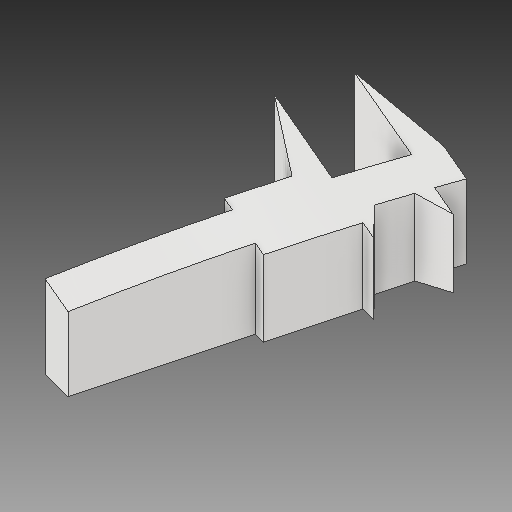
# Autodesk Inventor part: Team Pin Cad-Caliper
Saved by Autodesk Inventor 2017 (Build 210142000, 142)
## iProperties
Created: 2016-02-20
Part Number: Team Pin Cad-Caliper
Material: Generic
Document SubType Name: Modeling
Designer: RoksBot
Density: 1 g/cm^3
Appearance: White
Author: RoksBot
Autodesk Inventor part; units mm, degrees
ref_plane "YZ Plane" through (0, 0, 0) normal (1, 0, 0) x (0, 1, 0)
ref_plane "XZ Plane" through (0, 0, 0) normal (0, 1, 0) x (-1, 0, 0)
ref_plane "XY Plane" through (0, 0, 0) normal (0, 0, 1) x (1, 0, 0)
sketch "Sketch1" plane through (0, 0, 0) normal (0, 0, 1) x (1, 0, 0)
  line L0 (0, 0) -> (0, 8.6646) construction
  line L1 (20.9931, 1.27) -> (20.9931, 5.715)
  line L2 (20.9931, 5.715) -> (27.9781, 3.81)
  line L3 (27.9781, 3.81) -> (27.9781, 0)
  line L4 (27.9781, 0) -> (20.9931, 0)
  line L5 (20.9931, 1.27) -> (18.4531, 1.27)
  line L6 (18.4531, 1.27) -> (18.4531, 0)
  line L7 (18.4531, 0) -> (20.9931, 0)
  dimension "d0" = 20.9931
  dimension "d1" = 4.445
  dimension "d2" = 1.27
  dimension "d3" = 2.54
  dimension "d4" = 3.81
  dimension "d5" = 6.985
  constraints: 16 end point, 2 parallel, 2 perpendicular, 2 vertical, 1 horizontal, 1 horizontal alignment
  measures "d0" distance between parallel lines of L0 L1
  measures "d1" distance from line of L5 L1.end
  measures "d2" distance of L5.end L6.end
  measures "d3" distance between parallel lines of L1 L6
  measures "d4" distance of L2.end L3.end
  measures "d5" distance between parallel lines of L1 L3
revolve "Revolution1" add sketch "Sketch1" angle 360 about axis through (0, 0, 0) along (0, 1, 0)
sketch "Sketch2" plane through (0, 1.27, 0) normal (0, 1, 0) x (1, 0, 0)
  circle A0 centre (0, 0) radius 20.9931 projected
  circle A1 centre (0, 0) radius 27.9781 projected
  circle A2 centre (0, 0) radius 18.4531 projected
  line L0 (-4.2505, -7.1349) -> (4.1315, -7.1349) projected
  circle A3 centre (0, 0) radius 19.685 projected
  line L1 (-12.7595, -2.2222) -> (-12.7595, -29.7716) construction
  line L2 (12.6405, -2.2222) -> (12.6405, -30.8961) construction
  line L3 (-12.7549, -7.1349) -> (-31.6502, -7.1349) construction
  line L4 (0, 0) -> (17.3317, 30.0193) construction
  line L5 (-18.5741, 9.7833) -> (-25.4, 9.7833)
  line L6 (-18.8949, 9.1483) -> (-25.4, 9.1483)
  line L7 (-25.4, 9.1483) -> (-25.4, 9.7833)
  line L8 (-19.8553, -6.8174) -> (-25.4, -6.8174)
  line L9 (-25.4, -6.8174) -> (-25.4, -7.4524)
  line L10 (-25.4, -7.4524) -> (-19.6258, -7.4524)
  line L11 (0.1351, 9.4658) -> (-31.517, 9.4658) construction
  line L12 (-24.13, 9.1483) -> (-22.86, 6.9486)
  line L13 (-22.86, 6.9486) -> (-25.4, 6.9486)
  line L14 (-25.4, 6.9486) -> (-24.13, 9.1483)
  line L15 (-24.13, -6.8174) -> (-25.4, -4.6177)
  line L16 (-25.4, -4.6177) -> (-22.86, -4.6177)
  line L17 (-22.86, -4.6177) -> (-24.13, -6.8174)
  line L18 (-29.0818, 1.1654) -> (-16.5563, 1.1654) construction
  line L19 (-24.13, 7.6818) -> (-24.13, -5.3509) construction
  line L20 (-23.8125, 2.4354) -> (-24.4475, 2.4354)
  line L21 (-24.4475, 2.4354) -> (-24.4475, 6.9486)
  line L22 (-24.4475, 6.9486) -> (-23.8125, 6.9486)
  line L23 (-23.8125, 6.9486) -> (-23.8125, 2.4354)
  line L24 (-23.8125, 2.4354) -> (-24.4475, 6.9486) construction
  line L25 (-24.4475, 2.4354) -> (-23.8125, 6.9486) construction
  line L26 (-23.8125, -0.1046) -> (-24.4475, -0.1046)
  line L27 (-24.4475, -0.1046) -> (-24.4475, -4.6177)
  line L28 (-24.4475, -4.6177) -> (-23.8125, -4.6177)
  line L29 (-23.8125, -4.6177) -> (-23.8125, -0.1046)
  line L30 (-23.8125, -0.1046) -> (-24.4475, -4.6177) construction
  line L31 (-24.4475, -0.1046) -> (-23.8125, -4.6177) construction
  line L32 (-13.077, -16.4226) -> (-13.077, -23.7886)
  line L33 (-13.077, -23.7886) -> (-12.442, -23.7886)
  line L34 (-12.442, -23.7886) -> (-12.442, -16.9088)
  line L35 (12.323, -16.9957) -> (12.323, -23.7886)
  line L36 (12.323, -23.7886) -> (12.958, -23.7886)
  line L37 (12.958, -23.7886) -> (12.958, -16.5167)
  line L38 (-12.442, -22.5186) -> (-10.2423, -21.2486)
  line L39 (-10.2423, -21.2486) -> (-10.2423, -23.7886)
  line L40 (-10.2423, -23.7886) -> (-12.442, -22.5186)
  line L41 (12.323, -22.5186) -> (10.1233, -23.7886)
  line L42 (10.1233, -23.7886) -> (10.1233, -21.2486)
  line L43 (10.1233, -21.2486) -> (12.323, -22.5186)
  line L44 (-3.8695, -21.2486) -> (3.7505, -21.2486) construction
  line L45 (3.7505, -21.2486) -> (3.7505, -23.7886) construction
  line L46 (3.7505, -23.7886) -> (-3.8695, -23.7886) construction
  line L47 (-3.8695, -23.7886) -> (-3.8695, -21.2486) construction
  line L48 (-0.0595, -13.6296) -> (-0.0595, -32.797) construction
  line L49 (-10.2423, -22.5186) -> (10.1233, -22.5186) construction
  line L50 (-4.2505, -22.8361) -> (-10.2423, -22.8361)
  line L51 (-10.2423, -22.8361) -> (-10.2423, -22.2011)
  line L52 (-10.2423, -22.2011) -> (-4.2505, -22.2011)
  line L53 (-4.2505, -22.2011) -> (-4.2505, -22.8361)
  line L54 (-4.2505, -22.8361) -> (-10.2423, -22.2011) construction
  line L55 (-10.2423, -22.8361) -> (-4.2505, -22.2011) construction
  line L56 (4.1315, -22.2011) -> (10.1233, -22.2011)
  line L57 (10.1233, -22.2011) -> (10.1233, -22.8361)
  line L58 (10.1233, -22.8361) -> (4.1315, -22.8361)
  line L59 (4.1315, -22.8361) -> (4.1315, -22.2011)
  line L60 (4.1315, -22.2011) -> (10.1233, -22.8361) construction
  line L61 (10.1233, -22.2011) -> (4.1315, -22.8361) construction
  line L62 (10.2204, 18.3372) -> (11.1133, 19.8839)
  line L63 (11.1133, 19.8839) -> (11.6633, 19.5664)
  line L64 (11.6633, 19.5664) -> (10.7703, 18.0197)
  line L65 (12.8992, 20.8364) -> (18.6142, 20.8364) construction
  line L66 (18.6142, 20.8364) -> (18.6142, 18.2964) construction
  line L67 (18.6142, 18.2964) -> (12.8992, 18.2964) construction
  line L68 (12.8992, 18.2964) -> (12.8992, 20.8364) construction
  line L69 (11.1133, 19.8839) -> (12.8992, 19.8839)
  line L70 (12.8992, 19.8839) -> (12.8992, 19.2489)
  line L71 (12.8992, 19.2489) -> (11.1133, 19.2489)
  line L72 (11.1133, 19.2489) -> (11.1133, 19.8839)
  line L73 (11.1133, 19.8839) -> (12.8992, 19.2489) construction
  line L74 (12.8992, 19.8839) -> (11.1133, 19.2489) construction
  circle A4 centre (0, 0) radius 22.8981 construction
  line L75 (11.4654, -8.564) -> (6.3194, -8.564) projected
  spline S0 degree 2 poles (-4.3048, 23.0885) (-4.5009, 22.6771) (-4.9694, 22.2828) (-5.345, 22.1916) knots 0 0 0 1 2 2 2
  spline S1 degree 2 poles (-5.345, 22.1916) (-5.9856, 22.0361) (-6.5218, 22.4794) knots 0 0 0 1 1 1
  spline S2 degree 2 poles (-6.5218, 22.4794) (-7.071, 22.9258) (-7.2859, 23.8109) knots 0 0 0 1 1 1
  spline S3 degree 2 poles (-7.2859, 23.8109) (-7.5233, 24.7892) (-7.1789, 25.4155) knots 0 0 0 1 1 1
  spline S4 degree 2 poles (-7.1789, 25.4155) (-6.903, 25.9172) (-6.3614, 26.0486) knots 0 0 0 1 1 1
  spline S5 degree 2 poles (-6.3614, 26.0486) (-5.9392, 26.1511) (-5.6643, 26.0853) knots 0 0 0 1 1 1
  spline S6 degree 2 poles (-5.6643, 26.0853) (-5.3596, 26.0112) (-5.0862, 25.7107) knots 0 0 0 1 1 1
  spline S7 degree 2 poles (-5.0862, 25.7107) (-5.0278, 25.6478) (-5.0115, 25.5808) knots 0 0 0 1 1 1
  spline S8 degree 2 poles (-5.0115, 25.5808) (-4.9832, 25.4644) (-5.1191, 25.2618) (-5.2268, 25.2357) knots 0 0 0 1 2 2 2
  spline S9 degree 2 poles (-5.2268, 25.2357) (-5.3782, 25.1989) (-5.5051, 25.3408) knots 0 0 0 1 1 1
  spline S10 degree 2 poles (-5.5051, 25.3408) (-5.6451, 25.4856) (-5.8317, 25.5174) knots 0 0 0 1 1 1
  spline S11 degree 2 poles (-5.8317, 25.5174) (-5.9746, 25.5475) (-6.2279, 25.486) knots 0 0 0 1 1 1
  spline S12 degree 2 poles (-6.2279, 25.486) (-6.5569, 25.4061) (-6.7127, 25.0569) knots 0 0 0 1 1 1
  spline S13 degree 2 poles (-6.7127, 25.0569) (-6.906, 24.6338) (-6.7385, 23.9438) knots 0 0 0 1 1 1
  spline S14 degree 2 poles (-6.7385, 23.9438) (-6.5844, 23.309) (-5.8687, 22.6596) (-5.4727, 22.7557) knots 0 0 0 1 2 2 2
  spline S15 degree 2 poles (-5.4727, 22.7557) (-5.0447, 22.8596) (-4.8204, 23.3456) knots 0 0 0 1 1 1
  spline S16 degree 2 poles (-4.8204, 23.3456) (-4.7629, 23.4644) (-4.6377, 23.4948) knots 0 0 0 1 1 1
  spline S17 degree 2 poles (-4.6377, 23.4948) (-4.53, 23.521) (-4.3078, 23.393) (-4.2802, 23.2794) knots 0 0 0 1 2 2 2
  spline S18 degree 2 poles (-4.2802, 23.2794) (-4.2576, 23.1863) (-4.3048, 23.0885) knots 0 0 0 1 1 1
  spline S19 degree 2 poles (-2.5624, 23.1168) (-2.545, 22.971) (-2.7214, 22.7539) (-2.8582, 22.7376) knots 0 0 0 1 2 2 2
  spline S20 degree 2 poles (-2.8582, 22.7376) (-3.007, 22.7199) (-3.2201, 22.8877) (-3.2378, 23.0364) knots 0 0 0 1 2 2 2
  spline S21 degree 2 poles (-3.2378, 23.0364) (-3.254, 23.1733) (-3.087, 23.3923) (-2.9382, 23.41) knots 0 0 0 1 2 2 2
  spline S22 degree 2 poles (-2.9382, 23.41) (-2.8014, 23.4263) (-2.5783, 23.2507) (-2.5624, 23.1168) knots 0 0 0 1 2 2 2
  spline S23 degree 2 poles (1.6575, 23.2292) (1.6783, 23.1693) (1.6781, 23.1183) knots 0 0 0 1 1 1
  spline S24 degree 2 poles (1.6781, 23.1183) (1.6778, 22.9955) (1.4946, 22.8432) (1.3837, 22.8435) knots 0 0 0 1 2 2 2
  spline S25 degree 2 poles (1.3837, 22.8435) (1.189, 22.844) (1.1206, 23.024) knots 0 0 0 1 1 1
  line L76 (1.1206, 23.024) -> (0.9153, 23.5578)
  line L77 (0.9153, 23.5578) -> (-0.8255, 23.5626)
  line L78 (-0.8255, 23.5626) -> (-1.0307, 23.0328)
  spline S26 degree 2 poles (-1.0307, 23.0328) (-1.1001, 22.8503) (-1.2888, 22.8508) knots 0 0 0 1 1 1
  spline S27 degree 2 poles (-1.2888, 22.8508) (-1.4087, 22.8511) (-1.585, 23.0074) (-1.5847, 23.1272) knots 0 0 0 1 2 2 2
  spline S28 degree 2 poles (-1.5847, 23.1272) (-1.5846, 23.1812) (-1.5665, 23.2291) knots 0 0 0 1 1 1
  line L79 (-1.5665, 23.2291) -> (-0.2988, 26.5993)
  spline S29 degree 2 poles (-0.2988, 26.5993) (-0.2174, 26.8148) (0.0283, 26.8141) knots 0 0 0 1 1 1
  spline S30 degree 2 poles (0.0283, 26.8141) (0.28, 26.8135) (0.3484, 26.6245) knots 0 0 0 1 1 1
  line L80 (0.3484, 26.6245) -> (1.6575, 23.2292)
  line L81 (0.7221, 24.1366) -> (0.026, 25.9722)
  line L82 (0.026, 25.9722) -> (-0.6322, 24.1403)
  line L83 (-0.6322, 24.1403) -> (0.7221, 24.1366)
  spline S31 degree 2 poles (3.0603, 23.0562) (3.0422, 22.9105) (2.8189, 22.742) (2.6821, 22.7591) knots 0 0 0 1 2 2 2
  spline S32 degree 2 poles (2.6821, 22.7591) (2.5335, 22.7776) (2.3669, 22.9916) (2.3854, 23.1402) knots 0 0 0 1 2 2 2
  spline S33 degree 2 poles (2.3854, 23.1402) (2.4024, 23.277) (2.6172, 23.4495) (2.7658, 23.431) knots 0 0 0 1 2 2 2
  spline S34 degree 2 poles (2.7658, 23.431) (2.9026, 23.414) (3.077, 23.19) (3.0603, 23.0562) knots 0 0 0 1 2 2 2
  spline S35 degree 2 poles (7.2494, 23.9177) (6.9985, 22.8964) (6.3258, 22.4939) knots 0 0 0 1 1 1
  spline S36 degree 2 poles (6.3258, 22.4939) (5.7821, 22.1647) (5.1478, 22.3205) knots 0 0 0 1 1 1
  line L84 (5.1478, 22.3205) -> (4.1323, 22.5699)
  line L85 (4.1323, 22.5699) -> (5.0564, 26.3321)
  line L86 (5.0564, 26.3321) -> (6.069, 26.0834)
  spline S37 degree 2 poles (6.069, 26.0834) (6.6946, 25.9298) (7.047, 25.4051) knots 0 0 0 1 1 1
  spline S38 degree 2 poles (7.047, 25.4051) (7.4616, 24.7818) (7.2494, 23.9177) knots 0 0 0 1 1 1
  spline S39 degree 2 poles (6.7023, 24.052) (6.8474, 24.6427) (6.5732, 25.0587) knots 0 0 0 1 1 1
  spline S40 degree 2 poles (6.5732, 25.0587) (6.337, 25.416) (5.9267, 25.5167) knots 0 0 0 1 1 1
  line L87 (5.9267, 25.5167) -> (5.4641, 25.6304)
  line L88 (5.4641, 25.6304) -> (4.8173, 22.9971)
  line L89 (4.8173, 22.9971) -> (5.2857, 22.882)
  spline S41 degree 2 poles (5.2857, 22.882) (5.7047, 22.7791) (6.047, 22.9666) knots 0 0 0 1 1 1
  spline S42 degree 2 poles (6.047, 22.9666) (6.5215, 23.3159) (6.7023, 24.052) knots 0 0 0 1 1 1
  line L90 (-26.9128, 0.2129) -> (-27.3651, 0.2129)
  line L91 (-27.3651, 0.2129) -> (-27.3651, 0.7162)
  line L92 (-27.3651, 0.7162) -> (-26.9128, 0.7162)
  line L93 (-26.9128, 0.7162) -> (-26.9128, 0.2129)
  spline S43 degree 2 poles (-25.1468, 0.8613) (-25.1468, 0.5603) (-25.5281, 0.1728) (-25.8615, 0.1728) knots 0 0 0 1 2 2 2
  spline S44 degree 2 poles (-25.8615, 0.1728) (-26.0282, 0.1728) (-26.2891, 0.2685) (-26.3802, 0.3627) knots 0 0 0 1 2 2 2
  spline S45 degree 2 poles (-26.3802, 0.3627) (-26.4883, 0.4723) (-26.6041, 0.8196) (-26.6041, 1.062) knots 0 0 0 1 2 2 2
  spline S46 degree 2 poles (-26.6041, 1.062) (-26.6041, 1.3121) (-26.496, 1.7011) (-26.374, 1.8509) knots 0 0 0 1 2 2 2
  spline S47 degree 2 poles (-26.374, 1.8509) (-26.2583, 1.9929) (-25.8816, 2.1535) (-25.6238, 2.1535) knots 0 0 0 1 2 2 2
  spline S48 degree 2 poles (-25.6238, 2.1535) (-25.5296, 2.1535) (-25.3413, 2.1288) (-25.3073, 2.121) knots 0 0 0 1 2 2 2
  line L94 (-25.3073, 2.121) -> (-25.3073, 1.7474)
  line L95 (-25.3073, 1.7474) -> (-25.3413, 1.7474)
  spline S49 degree 2 poles (-25.3413, 1.7474) (-25.3752, 1.7644) (-25.5296, 1.8061) (-25.6284, 1.8061) knots 0 0 0 1 2 2 2
  spline S50 degree 2 poles (-25.6284, 1.8061) (-25.8523, 1.8061) (-26.0962, 1.5699) (-26.1255, 1.3507) knots 0 0 0 1 2 2 2
  spline S51 degree 2 poles (-26.1255, 1.3507) (-26.0313, 1.4109) (-25.8384, 1.4819) (-25.7164, 1.4819) knots 0 0 0 1 2 2 2
  spline S52 degree 2 poles (-25.7164, 1.4819) (-25.613, 1.4819) (-25.4324, 1.4263) (-25.3629, 1.3739) knots 0 0 0 1 2 2 2
  spline S53 degree 2 poles (-25.3629, 1.3739) (-25.2641, 1.2982) (-25.1468, 1.0528) (-25.1468, 0.8613) knots 0 0 0 1 2 2 2
  spline S54 degree 2 poles (-25.7041, 0.5742) (-25.667, 0.6205) (-25.6269, 0.7286) (-25.6269, 0.8382) knots 0 0 0 1 2 2 2
  spline S55 degree 2 poles (-25.6269, 0.8382) (-25.6269, 0.9308) (-25.6732, 1.0512) (-25.7149, 1.0867) knots 0 0 0 1 2 2 2
  spline S56 degree 2 poles (-25.7149, 1.0867) (-25.7581, 1.1238) (-25.8646, 1.15) (-25.9248, 1.15) knots 0 0 0 1 2 2 2
  spline S57 degree 2 poles (-25.9248, 1.15) (-25.9758, 1.15) (-26.0807, 1.1238) (-26.127, 1.1052) knots 0 0 0 1 2 2 2
  spline S58 degree 2 poles (-26.127, 1.1052) (-26.127, 1.0929) (-26.1301, 1.0342) (-26.1301, 0.9895) knots 0 0 0 1 2 2 2
  spline S59 degree 2 poles (-26.1301, 0.9895) (-26.1301, 0.8243) (-26.073, 0.6251) (-26.0282, 0.5742) knots 0 0 0 1 2 2 2
  spline S60 degree 2 poles (-26.0282, 0.5742) (-25.9958, 0.5325) (-25.9094, 0.497) (-25.8631, 0.497) knots 0 0 0 1 2 2 2
  spline S61 degree 2 poles (-25.8631, 0.497) (-25.8245, 0.497) (-25.7349, 0.5356) (-25.7041, 0.5742) knots 0 0 0 1 2 2 2
  spline S62 degree 2 poles (-23.5104, 0.8582) (-23.5104, 0.7085) (-23.6123, 0.4553) (-23.7126, 0.3642) knots 0 0 0 1 2 2 2
  spline S63 degree 2 poles (-23.7126, 0.3642) (-23.8129, 0.2732) (-24.0877, 0.1728) (-24.2884, 0.1728) knots 0 0 0 1 2 2 2
  spline S64 degree 2 poles (-24.2884, 0.1728) (-24.5015, 0.1744) (-24.8071, 0.2438) (-24.9075, 0.2886) knots 0 0 0 1 2 2 2
  line L96 (-24.9075, 0.2886) -> (-24.9075, 0.7039)
  line L97 (-24.9075, 0.7039) -> (-24.8643, 0.7039)
  spline S65 degree 2 poles (-24.8643, 0.7039) (-24.8272, 0.6838) (-24.7377, 0.6313) (-24.6651, 0.6035) knots 0 0 0 1 2 2 2
  spline S66 degree 2 poles (-24.6651, 0.6035) (-24.5972, 0.5773) (-24.4567, 0.5418) (-24.3718, 0.5418) knots 0 0 0 1 2 2 2
  spline S67 degree 2 poles (-24.3718, 0.5418) (-24.2977, 0.5418) (-24.1248, 0.5788) (-24.0723, 0.6282) knots 0 0 0 1 2 2 2
  spline S68 degree 2 poles (-24.0723, 0.6282) (-24.0337, 0.6668) (-23.9905, 0.761) (-23.9905, 0.8397) knots 0 0 0 1 2 2 2
  spline S69 degree 2 poles (-23.9905, 0.8397) (-23.9905, 0.9076) (-24.0461, 1.0034) (-24.0908, 1.0327) knots 0 0 0 1 2 2 2
  spline S70 degree 2 poles (-24.0908, 1.0327) (-24.1557, 1.0759) (-24.3409, 1.1006) (-24.4073, 1.1006) knots 0 0 0 1 2 2 2
  spline S71 degree 2 poles (-24.4073, 1.1006) (-24.5123, 1.1006) (-24.7114, 1.0666) (-24.784, 1.0481) knots 0 0 0 1 2 2 2
  line L98 (-24.784, 1.0481) -> (-24.8257, 1.0481)
  line L99 (-24.8257, 1.0481) -> (-24.8257, 2.1179)
  line L100 (-24.8257, 2.1179) -> (-23.5629, 2.1179)
  line L101 (-23.5629, 2.1179) -> (-23.5629, 1.7583)
  line L102 (-23.5629, 1.7583) -> (-24.3733, 1.7583)
  line L103 (-24.3733, 1.7583) -> (-24.3733, 1.4418)
  spline S72 degree 2 poles (-24.3733, 1.4418) (-24.3347, 1.4449) (-24.2282, 1.448) (-24.1989, 1.448) knots 0 0 0 1 2 2 2
  spline S73 degree 2 poles (-24.1989, 1.448) (-24.0615, 1.448) (-23.8299, 1.3924) (-23.7388, 1.3353) knots 0 0 0 1 2 2 2
  spline S74 degree 2 poles (-23.7388, 1.3353) (-23.6308, 1.2642) (-23.5104, 1.0281) (-23.5104, 0.8582) knots 0 0 0 1 2 2 2
  line L104 (-21.7752, 0.6575) -> (-22.033, 0.6575)
  line L105 (-22.033, 0.6575) -> (-22.033, 0.2083)
  line L106 (-22.033, 0.2083) -> (-22.4946, 0.2083)
  line L107 (-22.4946, 0.2083) -> (-22.4946, 0.6575)
  line L108 (-22.4946, 0.6575) -> (-23.3344, 0.6575)
  line L109 (-23.3344, 0.6575) -> (-23.3344, 1.0126)
  line L110 (-23.3344, 1.0126) -> (-22.51, 2.1179)
  line L111 (-22.51, 2.1179) -> (-22.033, 2.1179)
  line L112 (-22.033, 2.1179) -> (-22.033, 1.0003)
  line L113 (-22.033, 1.0003) -> (-21.7752, 1.0003)
  line L114 (-21.7752, 1.0003) -> (-21.7752, 0.6575)
  line L115 (-22.4946, 1.0003) -> (-22.4946, 1.6486)
  line L116 (-22.4946, 1.6486) -> (-22.9778, 1.0003)
  line L117 (-22.9778, 1.0003) -> (-22.4946, 1.0003)
  line L118 (-2.2979, -23.4704) -> (-3.5561, -23.4704)
  line L119 (-3.5561, -23.4704) -> (-3.5561, -23.1385)
  line L120 (-3.5561, -23.1385) -> (-3.1547, -23.1385)
  line L121 (-3.1547, -23.1385) -> (-3.1547, -22.1304)
  line L122 (-3.1547, -22.1304) -> (-3.5561, -22.1304)
  line L123 (-3.5561, -22.1304) -> (-3.5561, -21.8201)
  spline S75 degree 2 poles (-3.5561, -21.8201) (-3.4681, -21.8201) (-3.2937, -21.7969) (-3.2412, -21.7722) knots 0 0 0 1 2 2 2
  spline S76 degree 2 poles (-3.2412, -21.7722) (-3.181, -21.7413) (-3.113, -21.6379) (-3.1069, -21.5607) knots 0 0 0 1 2 2 2
  line L124 (-3.1069, -21.5607) -> (-2.69, -21.5607)
  line L125 (-2.69, -21.5607) -> (-2.69, -23.1385)
  line L126 (-2.69, -23.1385) -> (-2.2979, -23.1385)
  line L127 (-2.2979, -23.1385) -> (-2.2979, -23.4704)
  line L128 (-1.5029, -23.4704) -> (-1.9552, -23.4704)
  line L129 (-1.9552, -23.4704) -> (-1.9552, -22.9671)
  line L130 (-1.9552, -22.9671) -> (-1.5029, -22.9671)
  line L131 (-1.5029, -22.9671) -> (-1.5029, -23.4704)
  spline S77 degree 2 poles (0.2493, -22.5179) (0.2493, -22.7649) (0.1705, -23.1354) (0.0825, -23.2604) knots 0 0 0 1 2 2 2
  spline S78 degree 2 poles (0.0825, -23.2604) (-0.0039, -23.3839) (-0.2833, -23.5105) (-0.484, -23.5105) knots 0 0 0 1 2 2 2
  spline S79 degree 2 poles (-0.484, -23.5105) (-0.6862, -23.5105) (-0.9641, -23.3839) (-1.0521, -23.2573) knots 0 0 0 1 2 2 2
  spline S80 degree 2 poles (-1.0521, -23.2573) (-1.1401, -23.1323) (-1.2188, -22.7649) (-1.2188, -22.5179) knots 0 0 0 1 2 2 2
  spline S81 degree 2 poles (-1.2188, -22.5179) (-1.2188, -22.2647) (-1.1401, -21.9065) (-1.0506, -21.7769) knots 0 0 0 1 2 2 2
  spline S82 degree 2 poles (-1.0506, -21.7769) (-0.961, -21.6503) (-0.6785, -21.5268) (-0.484, -21.5268) knots 0 0 0 1 2 2 2
  spline S83 degree 2 poles (-0.484, -21.5268) (-0.2787, -21.5268) (-0.0039, -21.6564) (0.0841, -21.7846) knots 0 0 0 1 2 2 2
  spline S84 degree 2 poles (0.0841, -21.7846) (0.1705, -21.9096) (0.2493, -22.2786) (0.2493, -22.5179) knots 0 0 0 1 2 2 2
  spline S85 degree 2 poles (-0.2308, -22.5179) (-0.2308, -22.1643) (-0.3466, -21.8787) (-0.484, -21.8787) knots 0 0 0 1 2 2 2
  spline S86 degree 2 poles (-0.484, -21.8787) (-0.6214, -21.8787) (-0.7387, -22.1643) (-0.7387, -22.5194) knots 0 0 0 1 2 2 2
  spline S87 degree 2 poles (-0.7387, -22.5194) (-0.7387, -22.8683) (-0.6214, -23.1585) (-0.484, -23.1585) knots 0 0 0 1 2 2 2
  spline S88 degree 2 poles (-0.484, -23.1585) (-0.3482, -23.1585) (-0.2308, -22.8683) (-0.2308, -22.5179) knots 0 0 0 1 2 2 2
  spline S89 degree 2 poles (1.9181, -22.5179) (1.9181, -22.7649) (1.8393, -23.1354) (1.7513, -23.2604) knots 0 0 0 1 2 2 2
  spline S90 degree 2 poles (1.7513, -23.2604) (1.6649, -23.3839) (1.3855, -23.5105) (1.1848, -23.5105) knots 0 0 0 1 2 2 2
  spline S91 degree 2 poles (1.1848, -23.5105) (0.9826, -23.5105) (0.7047, -23.3839) (0.6167, -23.2573) knots 0 0 0 1 2 2 2
  spline S92 degree 2 poles (0.6167, -23.2573) (0.5287, -23.1323) (0.45, -22.7649) (0.45, -22.5179) knots 0 0 0 1 2 2 2
  spline S93 degree 2 poles (0.45, -22.5179) (0.45, -22.2647) (0.5287, -21.9065) (0.6182, -21.7769) knots 0 0 0 1 2 2 2
  spline S94 degree 2 poles (0.6182, -21.7769) (0.7078, -21.6503) (0.9903, -21.5268) (1.1848, -21.5268) knots 0 0 0 1 2 2 2
  spline S95 degree 2 poles (1.1848, -21.5268) (1.3901, -21.5268) (1.6649, -21.6564) (1.7529, -21.7846) knots 0 0 0 1 2 2 2
  spline S96 degree 2 poles (1.7529, -21.7846) (1.8393, -21.9096) (1.9181, -22.2786) (1.9181, -22.5179) knots 0 0 0 1 2 2 2
  spline S97 degree 2 poles (1.438, -22.5179) (1.438, -22.1643) (1.3222, -21.8787) (1.1848, -21.8787) knots 0 0 0 1 2 2 2
  spline S98 degree 2 poles (1.1848, -21.8787) (1.0474, -21.8787) (0.9301, -22.1643) (0.9301, -22.5194) knots 0 0 0 1 2 2 2
  spline S99 degree 2 poles (0.9301, -22.5194) (0.9301, -22.8683) (1.0474, -23.1585) (1.1848, -23.1585) knots 0 0 0 1 2 2 2
  spline S100 degree 2 poles (1.1848, -23.1585) (1.3206, -23.1585) (1.438, -22.8683) (1.438, -22.5179) knots 0 0 0 1 2 2 2
  spline S101 degree 2 poles (3.5869, -22.5179) (3.5869, -22.7649) (3.5081, -23.1354) (3.4202, -23.2604) knots 0 0 0 1 2 2 2
  spline S102 degree 2 poles (3.4202, -23.2604) (3.3337, -23.3839) (3.0543, -23.5105) (2.8536, -23.5105) knots 0 0 0 1 2 2 2
  spline S103 degree 2 poles (2.8536, -23.5105) (2.6514, -23.5105) (2.3735, -23.3839) (2.2855, -23.2573) knots 0 0 0 1 2 2 2
  spline S104 degree 2 poles (2.2855, -23.2573) (2.1975, -23.1323) (2.1188, -22.7649) (2.1188, -22.5179) knots 0 0 0 1 2 2 2
  spline S105 degree 2 poles (2.1188, -22.5179) (2.1188, -22.2647) (2.1975, -21.9065) (2.287, -21.7769) knots 0 0 0 1 2 2 2
  spline S106 degree 2 poles (2.287, -21.7769) (2.3766, -21.6503) (2.6591, -21.5268) (2.8536, -21.5268) knots 0 0 0 1 2 2 2
  spline S107 degree 2 poles (2.8536, -21.5268) (3.0589, -21.5268) (3.3337, -21.6564) (3.4217, -21.7846) knots 0 0 0 1 2 2 2
  spline S108 degree 2 poles (3.4217, -21.7846) (3.5081, -21.9096) (3.5869, -22.2786) (3.5869, -22.5179) knots 0 0 0 1 2 2 2
  spline S109 degree 2 poles (3.1068, -22.5179) (3.1068, -22.1643) (2.991, -21.8787) (2.8536, -21.8787) knots 0 0 0 1 2 2 2
  spline S110 degree 2 poles (2.8536, -21.8787) (2.7162, -21.8787) (2.5989, -22.1643) (2.5989, -22.5194) knots 0 0 0 1 2 2 2
  spline S111 degree 2 poles (2.5989, -22.5194) (2.5989, -22.8683) (2.7162, -23.1585) (2.8536, -23.1585) knots 0 0 0 1 2 2 2
  spline S112 degree 2 poles (2.8536, -23.1585) (2.9894, -23.1585) (3.1068, -22.8683) (3.1068, -22.5179) knots 0 0 0 1 2 2 2
  line L132 (14.3527, 18.6316) -> (13.0945, 18.6316)
  line L133 (13.0945, 18.6316) -> (13.0945, 18.9635)
  line L134 (13.0945, 18.9635) -> (13.4959, 18.9635)
  line L135 (13.4959, 18.9635) -> (13.4959, 19.9716)
  line L136 (13.4959, 19.9716) -> (13.0945, 19.9716)
  line L137 (13.0945, 19.9716) -> (13.0945, 20.2819)
  spline S113 degree 2 poles (13.0945, 20.2819) (13.1825, 20.2819) (13.357, 20.3051) (13.4094, 20.3298) knots 0 0 0 1 2 2 2
  spline S114 degree 2 poles (13.4094, 20.3298) (13.4697, 20.3606) (13.5376, 20.4641) (13.5438, 20.5412) knots 0 0 0 1 2 2 2
  line L138 (13.5438, 20.5412) -> (13.9606, 20.5412)
  line L139 (13.9606, 20.5412) -> (13.9606, 18.9635)
  line L140 (13.9606, 18.9635) -> (14.3527, 18.9635)
  line L141 (14.3527, 18.9635) -> (14.3527, 18.6316)
  line L142 (15.1477, 18.6316) -> (14.6954, 18.6316)
  line L143 (14.6954, 18.6316) -> (14.6954, 19.1349)
  line L144 (14.6954, 19.1349) -> (15.1477, 19.1349)
  line L145 (15.1477, 19.1349) -> (15.1477, 18.6316)
  spline S115 degree 2 poles (16.8814, 19.2769) (16.8814, 19.1272) (16.7795, 18.874) (16.6791, 18.7829) knots 0 0 0 1 2 2 2
  spline S116 degree 2 poles (16.6791, 18.7829) (16.5788, 18.6918) (16.304, 18.5915) (16.1033, 18.5915) knots 0 0 0 1 2 2 2
  spline S117 degree 2 poles (16.1033, 18.5915) (15.8903, 18.593) (15.5846, 18.6625) (15.4843, 18.7073) knots 0 0 0 1 2 2 2
  line L146 (15.4843, 18.7073) -> (15.4843, 19.1225)
  line L147 (15.4843, 19.1225) -> (15.5275, 19.1225)
  spline S118 degree 2 poles (15.5275, 19.1225) (15.5645, 19.1025) (15.6541, 19.05) (15.7266, 19.0222) knots 0 0 0 1 2 2 2
  spline S119 degree 2 poles (15.7266, 19.0222) (15.7946, 18.9959) (15.935, 18.9604) (16.0199, 18.9604) knots 0 0 0 1 2 2 2
  spline S120 degree 2 poles (16.0199, 18.9604) (16.094, 18.9604) (16.2669, 18.9975) (16.3194, 19.0469) knots 0 0 0 1 2 2 2
  spline S121 degree 2 poles (16.3194, 19.0469) (16.358, 19.0855) (16.4013, 19.1796) (16.4013, 19.2584) knots 0 0 0 1 2 2 2
  spline S122 degree 2 poles (16.4013, 19.2584) (16.4013, 19.3263) (16.3457, 19.422) (16.3009, 19.4514) knots 0 0 0 1 2 2 2
  spline S123 degree 2 poles (16.3009, 19.4514) (16.2361, 19.4946) (16.0508, 19.5193) (15.9844, 19.5193) knots 0 0 0 1 2 2 2
  spline S124 degree 2 poles (15.9844, 19.5193) (15.8795, 19.5193) (15.6803, 19.4853) (15.6078, 19.4668) knots 0 0 0 1 2 2 2
  line L148 (15.6078, 19.4668) -> (15.5661, 19.4668)
  line L149 (15.5661, 19.4668) -> (15.5661, 20.5366)
  line L150 (15.5661, 20.5366) -> (16.8289, 20.5366)
  line L151 (16.8289, 20.5366) -> (16.8289, 20.1769)
  line L152 (16.8289, 20.1769) -> (16.0184, 20.1769)
  line L153 (16.0184, 20.1769) -> (16.0184, 19.8604)
  spline S125 degree 2 poles (16.0184, 19.8604) (16.057, 19.8635) (16.1635, 19.8666) (16.1928, 19.8666) knots 0 0 0 1 2 2 2
  spline S126 degree 2 poles (16.1928, 19.8666) (16.3302, 19.8666) (16.5618, 19.811) (16.6529, 19.7539) knots 0 0 0 1 2 2 2
  spline S127 degree 2 poles (16.6529, 19.7539) (16.7609, 19.6829) (16.8814, 19.4467) (16.8814, 19.2769) knots 0 0 0 1 2 2 2
  spline S128 degree 2 poles (18.5502, 19.2769) (18.5502, 19.1272) (18.4483, 18.874) (18.3479, 18.7829) knots 0 0 0 1 2 2 2
  spline S129 degree 2 poles (18.3479, 18.7829) (18.2476, 18.6918) (17.9728, 18.5915) (17.7721, 18.5915) knots 0 0 0 1 2 2 2
  spline S130 degree 2 poles (17.7721, 18.5915) (17.5591, 18.593) (17.2534, 18.6625) (17.1531, 18.7073) knots 0 0 0 1 2 2 2
  line L154 (17.1531, 18.7073) -> (17.1531, 19.1225)
  line L155 (17.1531, 19.1225) -> (17.1963, 19.1225)
  spline S131 degree 2 poles (17.1963, 19.1225) (17.2333, 19.1025) (17.3229, 19.05) (17.3954, 19.0222) knots 0 0 0 1 2 2 2
  spline S132 degree 2 poles (17.3954, 19.0222) (17.4634, 18.9959) (17.6038, 18.9604) (17.6887, 18.9604) knots 0 0 0 1 2 2 2
  spline S133 degree 2 poles (17.6887, 18.9604) (17.7628, 18.9604) (17.9358, 18.9975) (17.9882, 19.0469) knots 0 0 0 1 2 2 2
  spline S134 degree 2 poles (17.9882, 19.0469) (18.0268, 19.0855) (18.0701, 19.1796) (18.0701, 19.2584) knots 0 0 0 1 2 2 2
  spline S135 degree 2 poles (18.0701, 19.2584) (18.0701, 19.3263) (18.0145, 19.422) (17.9697, 19.4514) knots 0 0 0 1 2 2 2
  spline S136 degree 2 poles (17.9697, 19.4514) (17.9049, 19.4946) (17.7196, 19.5193) (17.6532, 19.5193) knots 0 0 0 1 2 2 2
  spline S137 degree 2 poles (17.6532, 19.5193) (17.5483, 19.5193) (17.3491, 19.4853) (17.2766, 19.4668) knots 0 0 0 1 2 2 2
  line L156 (17.2766, 19.4668) -> (17.2349, 19.4668)
  line L157 (17.2349, 19.4668) -> (17.2349, 20.5366)
  line L158 (17.2349, 20.5366) -> (18.4977, 20.5366)
  line L159 (18.4977, 20.5366) -> (18.4977, 20.1769)
  line L160 (18.4977, 20.1769) -> (17.6872, 20.1769)
  line L161 (17.6872, 20.1769) -> (17.6872, 19.8604)
  spline S138 degree 2 poles (17.6872, 19.8604) (17.7258, 19.8635) (17.8323, 19.8666) (17.8616, 19.8666) knots 0 0 0 1 2 2 2
  spline S139 degree 2 poles (17.8616, 19.8666) (17.999, 19.8666) (18.2306, 19.811) (18.3217, 19.7539) knots 0 0 0 1 2 2 2
  spline S140 degree 2 poles (18.3217, 19.7539) (18.4298, 19.6829) (18.5502, 19.4467) (18.5502, 19.2769) knots 0 0 0 1 2 2 2
  point P0 (-10.4828, 14.7667)
  point P1 (-24.13, 4.692)
  point P2 (-24.13, -2.3611)
  point P3 (-10.9755, -22.5186)
  point P4 (10.8565, -22.5186)
  point P5 (-3.8695, -22.5186)
  point P6 (-0.0595, -23.7886)
  point P7 (-7.2464, -22.5186)
  point P8 (7.1274, -22.5186)
  point P9 (12.0063, 19.5664)
  point P10 (12.0063, 19.5664)
  point P11 (18.6142, 19.5664)
  dimension "d60" = 0.635
  dimension "d7" = 39.37
  dimension "d9" = 25.4
  dimension "d11" = 0.635
  dimension "d13" = 25.4
  dimension "d14" = 0.635
  dimension "d15" = 0.3175
  dimension "d16" = 16.6007
  dimension "d17" = 0.3175
  dimension "d18" = 2.54
  dimension "d19" = 1.27
  dimension "d20" = 1.27
  dimension "d21" = 0.635
  dimension "d22" = 0.3175
  dimension "d23" = 7.366
  dimension "d24" = 0.3175
  dimension "d25" = 2.54
  dimension "d26" = 7.62
  dimension "d27" = 2.54
  dimension "d28" = 0.635
  dimension "d29" = 0.381
  dimension "d30" = 0.381
  dimension "d31" = 0.635
  dimension "d32" = 0.3175
  dimension "d33" = 5.715
  dimension "d34" = 2.54
  dimension "d35" = 27.94
  dimension "d36" = 0.635
  dimension "d38" = 60
  dimension "d39" = 1.905
  constraints: 132 end point, 16 midpoint, 16 point on line, 14 perpendicular, 13 horizontal, 12 parallel, 8 vertical, 5 equal length, 5 horizontal alignment, 3 vertical alignment, 1 centre point, 1 coincident, 1 collinear, 50 other
  measures "d7" diameter of A3
  measures "d9" distance between parallel lines of L2 L1
  measures "d11" distance between parallel lines of L6 L5
  measures "d13" horizontal distance of A1.centre L5.end
  measures "d14" distance between parallel lines of L10 L8
  measures "d15" distance between parallel lines of L10 L3
  measures "d16" distance from line of L11.start L0
  measures "d17" distance between parallel lines of L11 L5
  measures "d18" distance of L12.end L13.end
  measures "d19" distance between parallel lines of L18 L20
  measures "d20" distance between parallel lines of L18 L26
  measures "d21" distance of L32.end L33.end
  measures "d22" distance between parallel lines of L1 L32
  measures "d23" distance of L32.start L32.end
  measures "d24" distance between parallel lines of L2 L35
  measures "d25" distance of L38.end L39.end
  measures "d26" distance of L45.end L46.end
  measures "d27" distance of L44.end L45.end
  measures "d28" distance of L52.end L50.start
  measures "d29" distance between parallel lines of L47 L53
  measures "d30" distance between parallel lines of L45 L59
  measures "d31" distance of L62.end L63.end
  measures "d32" distance between parallel lines of L4 L62
  measures "d33" distance of L65.start L65.end
  measures "d34" distance of L65.end L66.end
  measures "d35" distance of A1.centre L65.end
  measures "d36" distance of L69.end L70.end
  measures "d38" angle of L0 L4
extrude "Extrusion1" cut sketch "Sketch2" along normal through all contours L41 L42 L43 | L38 L39 L40 | L15 L16 L17 | L12 L13 L14 | A0 L62 L72 L71 L64 | L37 L36 L35 A0 | L71 L72 L63 L64 | L64 L63 L69 L70 L71 | A0 L6 L7 L5 | L34 L33 L32 A0 | A0 L10 L9 L8 | L58 L59 L56 L42 | L52 L53 L50 L39 | L23 L20 L21 L13 | L27 L26 L29 L16 | S0 S1 S2 S3 S4 S5 S6 S7 S8 S9 S10 S11 S12 S13 S14 S15 S16 S17 S18 | S19 S20 S21 S22 | S23 S24 S25 L76 L77 L78 S26 S27 S28 L79 S29 S30 L80 | S31 S32 S33 S34 | S35 S36 L84 L85 L86 S37 S38 | L90 L91 L92 L93 | S43 S44 S45 S46 S47 S48 L94 L95 S49 S50 S51 S52 S53 | S62 S63 S64 L96 L97 S65 S66 S67 S68 S69 S70 S71 L98 L99 L100 L101 L102 L103 S72 S73 S74 | L104 L105 L106 L107 L108 L109 L110 L111 L112 L113 L114 | L118 L119 L120 L121 L122 L123 S75 S76 L124 L125 L126 L127 | L128 L129 L130 L131 | S77 S78 S79 S80 S81 S82 S83 S84 | S89 S90 S91 S92 S93 S94 S95 S96 | S101 S102 S103 S104 S105 S106 S107 S108 | L132 L133 L134 L135 L136 L137 S113 S114 L138 L139 L140 L141 | L142 L143 L144 L145 | S115 S116 S117 L146 L147 S118 S119 S120 S121 S122 S123 S124 L148 L149 L150 L151 L152 L153 S125 S126 S127 | S128 S129 S130 L154 L155 S131 S132 S133 S134 S135 S136 S137 L156 L157 L158 L159 L160 L161 S138 S139 S140
sketch "Sketch3" plane through (-25.4, 1.27, -9.7833) normal (0, 1, 0) x (1, 0, 0)
  circle A0 centre (25.4, -9.7833) radius 18.415 projected
  circle A1 centre (25.4, -9.7833) radius 19.685 projected
  circle A2 centre (25.4, -9.7833) radius 27.9781 projected
  line L0 (48.8767, -22.6479) -> (52.1637, -10.3806)
  line L1 (52.1637, -10.3806) -> (50.937, -10.0519)
  line L2 (50.937, -10.0519) -> (47.65, -22.3192)
  line L3 (47.65, -22.3192) -> (48.8767, -22.6479)
  line L4 (48.8767, -22.6479) -> (50.937, -10.0519) construction
  line L5 (52.1637, -10.3806) -> (47.65, -22.3192) construction
  line L6 (49.5872, -13.3717) -> (48.7655, -16.4385)
  line L7 (48.7655, -16.4385) -> (50.8509, -16.9973)
  line L8 (50.8509, -16.9973) -> (51.6727, -13.9305)
  line L9 (51.6727, -13.9305) -> (49.5872, -13.3717)
  line L10 (49.5872, -13.3717) -> (50.8509, -16.9973) construction
  line L11 (48.7655, -16.4385) -> (51.6727, -13.9305) construction
  line L12 (50.937, -10.0519) -> (47.6072, -10.2115)
  line L13 (47.6072, -10.2115) -> (50.674, -11.0333)
  line L14 (49.5872, -13.3717) -> (46.9498, -12.665)
  line L15 (46.9498, -12.665) -> (49.3243, -14.3531)
  line L16 (51.9007, -11.362) -> (52.8821, -11.625)
  line L17 (52.8821, -11.625) -> (51.7364, -11.9754)
  line L18 (25.4, -9.7833) -> (37.7185, -9.7833) construction
  line L19 (51.6727, -13.9305) -> (52.2247, -14.0784)
  line L20 (52.2247, -14.0784) -> (51.4077, -13.2021)
  line L21 (51.4077, -13.2021) -> (51.2433, -13.8154) construction
  point P0 (49.9068, -16.3499)
  point P1 (50.2191, -15.1845)
  dimension "d42" = 3.175
  dimension "d43" = 3.175
  dimension "d44" = 1.016
  dimension "d45" = 1.27
  dimension "d46" = 1.016
  dimension "d47" = 1.016
  dimension "d49" = 0.635
  dimension "d50" = 3.175
  dimension "d51" = 12.7
  dimension "d52" = 2.159
  dimension "d53" = 2.54
  dimension "d54" = 25.4
  dimension "d55" = 0.635
  dimension "d56" = 25.5384
  dimension "d57" = 25.5384
  dimension "d58" = 15
  dimension "d59" = 1.016
  dimension "d60" = 0.635
  constraints: 44 end point, 10 point on line, 6 parallel, 4 midpoint, 3 perpendicular, 1 horizontal
  measures "d42" distance from line of L2 L12.end
  measures "d43" distance from line of L2 L14.end
  measures "d44" distance of L6.start L15.end
  measures "d45" distance between parallel lines of L0 L2
  measures "d46" distance of L1.end L13.end
  measures "d47" distance of L16.start L16.end
  measures "d49" distance of L16.start L17.end
  measures "d50" distance of L7.end L8.end
  measures "d51" distance between parallel lines of L3 L1
  measures "d52" distance between parallel lines of L8 L6
  measures "d53" distance between parallel lines of L14 L13
  measures "d54" distance of point (25.4, -9.783) point (50.219, -15.185)
  measures "d55" distance from line of L0 point (50.219, -15.185)
  measures "d56" distance of A0.centre L1.end
  measures "d57" distance of A0.centre L2.end
  measures "d58" angle of L9 L18
  measures "d59" distance from line of L0 L19.end
  measures "d60" distance from line of L9 L20.end
extrude "Extrusion2" cut sketch "Sketch3" along normal through all contours L0 L9 L2 L1 | L20 L19 L9 L0 | L0 L16 L17 | L9 L8 L7 L0 | L0 L7 L2 L9 | L0 L3 L2 L7 | L2 L7 L6 L9 | L13 L12 L2 | L6 L15 L14 keep common part
equation "\"d15\" = 0.5 * d14"
equation "\"d17\" = 0.5 * d11"
equation "\"d22\" = 0.5 * d21"
equation "\"d24\" = d22"
equation "\"d32\" = 0.5 * d31"
body "Solid1"
